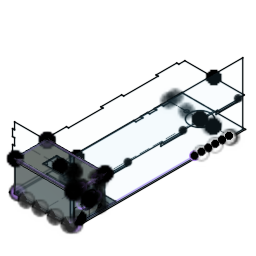
Stepper Bodies (Autodesk Fusion 360 design; units mm, degrees)
Autodesk Fusion 360 part; units mm, degrees
(part 1 of 5)
sketch "Sketch1" plane through (0, 0, 0) normal (0, 0, 1) x (1, 0, 0)
  line L0 (0, 0) -> (80, 0)
  line L1 (80, 0) -> (80, 42.25)
  line L2 (80, 42.25) -> (0, 42.25)
  line L3 (0, 42.25) -> (0, 0)
  line L4 (0, 0) -> (-2, 0) construction
  line L5 (-2, 0) -> (-2, -2) construction
  line L6 (-2, -2) -> (0, -2) construction
  line L7 (0, -2) -> (0, 0) construction
  line L8 (-2, -2) -> (82, -2)
  line L9 (82, -2) -> (82, 44.25)
  line L10 (82, 44.25) -> (-2, 44.25)
  line L11 (-2, 44.25) -> (-2, -2)
  line L12 (-2, 44.25) -> (82, 44.25) construction
  line L13 (82, 44.25) -> (82, 59.25)
  line L14 (82, 59.25) -> (-2, 59.25)
  line L15 (-2, 59.25) -> (-2, 44.25)
  line L16 (-2, 44.25) -> (82, 44.25) construction
  line L17 (82, 44.25) -> (82, 51.75) construction
  line L18 (82, 51.75) -> (-2, 51.75) construction
  line L19 (-2, 51.75) -> (-2, 44.25) construction
  circle A0 centre (40, 51.75) radius 2.5
  line L20 (40, 51.75) -> (-2, 51.75) construction
  circle A1 centre (19, 51.75) radius 2.5
  line L21 (40, 59.25) -> (40, 44.25) construction
  circle A2 centre (61, 51.75) radius 2.5
  dimension "d9" = 80
  dimension "d10" = 42.25
  dimension "d11" = 2
  dimension "d12" = 2
  dimension "d13" = 84
  dimension "d14" = 46.25
  dimension "d15" = 84
  dimension "d16" = 15
  dimension "d17" = 5
  dimension "d18" = 5
  constraint horizontal L0
  constraint vertical L1
  constraint horizontal L2
  constraint vertical L3
  constraint coincident L0.start L3.end
  constraint horizontal L4
  constraint vertical L5
  constraint horizontal L6
  constraint vertical L7
  constraint horizontal L8
  constraint vertical L9
  constraint horizontal L10
  constraint vertical L11
  constraint horizontal L12
  constraint vertical L13
  constraint horizontal L14
  constraint vertical L15
  constraint horizontal L16
  constraint vertical L17
  constraint horizontal L18
  constraint vertical L19
  constraint midpoint L13 L17.end
  constraint midpoint L18 A0.centre
  constraint coincident A0.centre L20.start
  constraint midpoint L20 A1.centre
  constraint midpoint L14 L21.start
  constraint midpoint L16 L21.end
  constraint symmetric A1 L21 A2
  measures "d9" distance of L0.start L0.end
  measures "d10" distance of L0.start L2.end
  measures "d11" distance of L0.start L4.end
  measures "d12" distance of L0.start L6.end
  measures "d13" distance of L5.end L8.end
  measures "d14" distance of L5.end L10.end
  measures "d15" distance of L10.end L9.end
  measures "d16" distance of L10.end L14.end
  measures "d17" diameter of A0
  measures "d18" diameter of A1
extrude "Extrude1" add sketch "Sketch1" along normal blind 42.25 contours L8 L9 L10 L11 makes body 1
extrude "Extrude2" add sketch "Sketch1" against normal blind 2 contours L0 L1 L2 L3 | L8 L9 L10 L11 | L10 L13 L14 L15 bodies 1
sketch "Sketch2" plane through (82, 0, 0) normal (1, 0, 0) x (0, 1, 0)
  line L0 (44.25, 0) -> (44.25, 42.25)
  line L1 (44.25, 42.25) -> (-2, 42.25)
  line L2 (-2, 42.25) -> (-2, -2)
  line L3 (-2, -2) -> (59.25, -2)
  line L4 (59.25, -2) -> (59.25, 0)
  line L5 (59.25, 0) -> (44.25, 0)
  line L6 (0, 0) -> (6, 0) construction
  line L7 (6, 0) -> (6, 6) construction
  line L8 (6, 6) -> (0, 6) construction
  line L9 (0, 6) -> (0, 0) construction
  circle A0 centre (6, 6) radius 2
  line L10 (0, 0) -> (21.125, 0) construction
  line L11 (21.125, 0) -> (21.125, 21.125) construction
  line L12 (21.125, 21.125) -> (0, 21.125) construction
  line L13 (0, 21.125) -> (0, 0) construction
  circle A1 centre (36.25, 6) radius 2
  circle A2 centre (6, 36.25) radius 2
  circle A3 centre (36.25, 36.25) radius 2
  circle A4 centre (21.125, 21.125) radius 11
  line L14 (10.125, 21.125) -> (10.125, 42.25)
  line L15 (32.125, 21.125) -> (32.125, 42.25)
  dimension "d24" = 6
  dimension "d25" = 6
  dimension "d26" = 4
  dimension "d27" = 21.125
  dimension "d28" = 21.125
  dimension "d32" = 22
  dimension "d33" = 21.125
  constraint horizontal L6
  constraint vertical L7
  constraint horizontal L8
  constraint vertical L9
  constraint coincident L6.start L9.end
  constraint coincident L7.end L8.start
  constraint horizontal L10
  constraint vertical L11
  constraint horizontal L12
  constraint vertical L13
  constraint symmetric A0 L11 A1
  constraint symmetric A0 L12 A2
  constraint symmetric L12 A1 A3
  constraint coincident L11.end L12.start
  constraint perpendicular L1 L14
  constraint coincident L12 L14.start
  constraint tangent A4 L14
  constraint symmetric L11 L14.start L15.start
  constraint symmetric L11 L14.end L15.end
  measures "d24" distance of L6.start L6.end
  measures "d25" distance of L6.start L8.end
  measures "d26" diameter of A0
  measures "d27" distance of L6.start L10.end
  measures "d28" distance of L6.start L12.end
  measures "d32" diameter of A4
  measures "d33" distance of L14.start L14.end
extrude "Extrude4" cut sketch "Sketch2" against normal blind 100 contours L1 A4 L14 L15 | A4 bodies 1
sketch "Sketch5" plane through (0, 0, 0) normal (0, 0, 1) x (1, 0, 0)
  line L0 (0, 0) -> (-6, 0) construction
  line L1 (-6, 0) -> (-6, -6) construction
  line L2 (-6, -6) -> (0, -6) construction
  line L3 (0, -6) -> (0, 0) construction
  line L4 (86, 244) -> (-6, 244)
  line L5 (-6, 244) -> (40, 244) construction
  line L6 (40, 244) -> (40, 224) construction
  line L7 (40, 224) -> (-6, 224) construction
  line L8 (-6, 224) -> (-6, 244) construction
  circle A0 centre (40, 224) radius 15
  circle A1 centre (19, 51.75) radius 2.5
  circle A2 centre (40, 51.75) radius 2.5
  circle A3 centre (61, 51.75) radius 2.5
  line L9 (-6, 224) -> (86, 224) construction
  line L10 (55, 224) -> (57, 224) construction
  circle A4 centre (59.5, 224) radius 2.5
  line L11 (57, 226.5) -> (57, 221.5) construction
  circle A5 centre (20.5, 224) radius 2.5
  circle A6 centre (19, 51.75) radius 2.5
  circle A7 centre (40, 51.75) radius 2.5
  circle A8 centre (61, 51.75) radius 2.5
  line L12 (-6, 244) -> (-6, 234) construction
  line L13 (-6, 224) -> (-3, 224)
  line L14 (-3, 224) -> (-3, 214)
  line L15 (-3, 214) -> (-6, 214)
  line L16 (-6, 244) -> (-6, 224)
  line L17 (-6, 214) -> (-6, 204) construction
  line L18 (-6, 204) -> (-3, 204)
  line L19 (-3, 204) -> (-3, 194)
  line L20 (-3, 194) -> (-6, 194)
  line L21 (-6, 214) -> (-6, 204)
  line L22 (-6, 194) -> (-6, 184) construction
  line L23 (-6, 184) -> (-3, 184)
  line L24 (-3, 184) -> (-3, 174)
  line L25 (-3, 174) -> (-6, 174)
  line L26 (-6, 194) -> (-6, 184)
  line L27 (-6, 174) -> (-6, -6)
  line L28 (-6, -6) -> (4, -6) construction
  line L29 (14, -6) -> (14, -3)
  line L30 (14, -3) -> (4, -3)
  line L31 (4, -3) -> (4, -6)
  line L32 (-6, -6) -> (4, -6)
  line L33 (14, -6) -> (24, -6) construction
  line L34 (34, -6) -> (34, -3)
  line L35 (34, -3) -> (24, -3)
  line L36 (24, -3) -> (24, -6)
  line L37 (14, -6) -> (24, -6)
  line L38 (40, 244) -> (40, -6) construction
  line L39 (76, -3) -> (76, -6)
  line L40 (66, -3) -> (76, -3)
  line L41 (66, -6) -> (66, -3)
  line L42 (56, -3) -> (56, -6)
  line L43 (46, -3) -> (56, -3)
  line L44 (46, -6) -> (46, -3)
  line L45 (34, -6) -> (46, -6)
  line L46 (56, -6) -> (66, -6)
  line L47 (76, -6) -> (86, -6)
  line L48 (83, 224) -> (83, 214)
  line L49 (83, 214) -> (86, 214)
  line L50 (86, 224) -> (83, 224)
  line L51 (86, 204) -> (83, 204)
  line L52 (83, 204) -> (83, 194)
  line L53 (83, 194) -> (86, 194)
  line L54 (86, 184) -> (83, 184)
  line L55 (83, 184) -> (83, 174)
  line L56 (83, 174) -> (86, 174)
  line L57 (86, 224) -> (86, 244)
  line L58 (86, 204) -> (86, 214)
  line L59 (86, -6) -> (86, 174)
  line L60 (86, 184) -> (86, 194)
  point P0 (40, 224)
  dimension "d40" = 6
  dimension "d41" = 6
  dimension "d44" = 92
  dimension "d45" = 250
  dimension "d47" = 46
  dimension "d48" = 20
  dimension "d50" = 30
  dimension "d52" = 2
  dimension "d53" = 5
  dimension "d54" = 5
  dimension "d55" = 5
  dimension "d56" = 5
  dimension "d57" = 5
  dimension "d60" = 10
  dimension "d61" = 3
  dimension "d62" = 10
  dimension "d63" = 10
  dimension "d64" = 3
  dimension "d65" = 10
  dimension "d92" = 10
  dimension "d93" = 3
  dimension "d94" = 10
  dimension "d95" = 10
  dimension "d96" = 10
  dimension "d97" = 3
  dimension "d98" = 10
  dimension "d99" = 10
  dimension "d100" = 3
  constraint horizontal L0
  constraint vertical L1
  constraint horizontal L2
  constraint vertical L3
  constraint coincident L0.start L3.end
  constraint horizontal L32
  constraint vertical L59
  constraint horizontal L4
  constraint vertical L16
  constraint horizontal L5
  constraint vertical L6
  constraint horizontal L7
  constraint vertical L8
  constraint coincident P0 L6.end
  constraint midpoint L9 P0
  constraint perpendicular L9 L57
  constraint coincident A0 L10.start
  constraint coincident L9 L10.start
  constraint perpendicular L10 L57
  constraint coincident L9 A4.centre
  constraint midpoint L10.end L11
  constraint perpendicular L10 L11
  constraint tangent A4 L11
  constraint symmetric L6 A4 A5
  constraint concentric A1 A6
  constraint concentric A2 A7
  constraint concentric A3 A8
  constraint perpendicular L7 L12
  constraint horizontal L13
  constraint vertical L14
  constraint horizontal L15
  constraint collinear L16 L21
  constraint perpendicular L15 L17
  constraint horizontal L18
  constraint vertical L19
  constraint horizontal L20
  constraint collinear L21 L26
  constraint perpendicular L20 L22
  constraint horizontal L23
  constraint vertical L24
  constraint horizontal L25
  constraint collinear L26 L27
  constraint perpendicular L28 L59
  constraint vertical L29
  constraint horizontal L30
  constraint vertical L31
  constraint collinear L32 L37
  constraint vertical L34
  constraint horizontal L35
  constraint vertical L36
  constraint collinear L37 L45
  constraint coincident L38.end L45
  constraint perpendicular L38 L45
  constraint symmetric L28.end L38 L39.end
  constraint symmetric L29.start L38 L41.start
  constraint symmetric L29.end L38 L40.start
  constraint symmetric L30.end L38 L39.start
  constraint symmetric L33.end L38 L42.end
  constraint symmetric L34.start L38 L44.start
  constraint symmetric L34.end L38 L43.start
  constraint symmetric L35.end L38 L42.start
  constraint collinear L45 L46
  constraint collinear L46 L47
  constraint symmetric L7.end L38 L9.end
  constraint symmetric L13.end L38 L48.start
  constraint symmetric L14.end L38 L48.end
  constraint symmetric L15.end L38 L49.end
  constraint symmetric L17.end L38 L51.start
  constraint symmetric L18.end L38 L51.end
  constraint symmetric L19.end L38 L52.end
  constraint symmetric L20.end L38 L53.end
  constraint symmetric L22.end L38 L54.start
  constraint symmetric L23.end L38 L54.end
  constraint symmetric L24.end L38 L55.end
  constraint symmetric L25.end L38 L56.end
  constraint collinear L57 L58
  constraint collinear L58 L60
  constraint collinear L59 L60
  measures "d40" distance of L0.start L0.end
  measures "d41" distance of L0.start L2.end
  measures "d44" distance of L1.end L47.end
  measures "d45" distance of L1.end L4.end
  measures "d47" distance of L4.end L5.end
  measures "d48" distance of L4.end L7.end
  measures "d50" diameter of A0
  measures "d52" distance of L10.start L10.end
  measures "d53" diameter of A4
  measures "d54" distance of L11.start L11.end
  measures "d55" diameter of A6
  measures "d56" diameter of A7
  measures "d57" diameter of A8
  measures "d60" distance of L4.end L12.end
  measures "d61" distance of L7.end L13.end
  measures "d62" distance of L7.end L15.end
  measures "d63" distance of L15.end L17.end
  measures "d64" distance of L17.end L18.end
  measures "d65" distance of L17.end L20.end
  measures "d92" distance of L20.end L22.end
  measures "d93" distance of L22.end L23.end
  measures "d94" distance of L22.end L25.end
  measures "d95" distance of L1.end L28.end
  measures "d96" distance of L28.end L29.start
  measures "d97" distance of L28.end L30.end
  measures "d98" distance of L29.start L33.end
  measures "d99" distance of L33.end L34.start
  measures "d100" distance of L33.end L35.end
ref_plane "WorkPlane2" through (40, 21.125, 42.25) normal (0, 0, 1) x (1, 0, 0)
sketch "Sketch6" plane through (0, 0, 42.25) normal (0, 0, 1) x (1, 0, 0)
  line L0 (-2, 44.25) -> (82, 44.25)
  line L1 (-2, 44.25) -> (-2, -2)
  line L2 (-2, -2) -> (82, -2)
  line L3 (82, 10.125) -> (82, 32.125)
  line L4 (82, -2) -> (82, 44.25)
  line L5 (82, 4) -> (82, 8)
  line L6 (-2, 44.25) -> (-3, 44.25) construction
  line L7 (-3, 44.25) -> (-3, 45.25) construction
  line L8 (-3, 45.25) -> (-2, 45.25) construction
  line L9 (-2, 45.25) -> (-2, 44.25) construction
  line L10 (-2, -2) -> (-3, -2) construction
  line L11 (-3, -2) -> (-3, -3) construction
  line L12 (-3, -3) -> (-2, -3) construction
  line L13 (-2, -3) -> (-2, -2) construction
  line L14 (82, -2) -> (83, -2) construction
  line L15 (83, -2) -> (83, -3) construction
  line L16 (83, -3) -> (82, -3) construction
  line L17 (82, -3) -> (82, -2) construction
  line L18 (82, 44.25) -> (83, 44.25) construction
  line L19 (83, 44.25) -> (83, 45.25) construction
  line L20 (83, 45.25) -> (82, 45.25) construction
  line L21 (82, 45.25) -> (82, 44.25) construction
  line L22 (-3, 45.25) -> (83, 45.25)
  line L23 (83, 45.25) -> (83, -3)
  line L24 (83, -3) -> (-3, -3)
  line L25 (-3, -3) -> (-3, 45.25)
  line L26 (-2, 44.25) -> (82, 44.25)
  line L27 (82, 44.25) -> (82, -2)
  line L28 (82, -2) -> (-2, -2)
  line L29 (-2, -2) -> (-2, 44.25)
  line L30 (-2, 21.125) -> (82, 21.125) construction
  line L31 (40, 44.25) -> (40, -2) construction
  line L32 (55, 31.125) -> (25, 31.125)
  line L33 (25, 31.125) -> (25, 11.125)
  line L34 (25, 11.125) -> (55, 11.125)
  line L35 (55, 11.125) -> (55, 31.125)
  line L36 (55, 31.125) -> (25, 11.125) construction
  line L37 (25, 31.125) -> (55, 11.125) construction
  point P0 (82, 36.25)
  point P1 (82, 6)
  point P2 (40, 21.125)
  dimension "d68" = 1
  dimension "d69" = 1
  dimension "d70" = 1
  dimension "d71" = 1
  dimension "d72" = 1
  dimension "d73" = 1
  dimension "d74" = 1
  dimension "d75" = 1
  dimension "d86" = 30
  dimension "d87" = 20
  constraint horizontal L6
  constraint vertical L7
  constraint horizontal L8
  constraint vertical L9
  constraint coincident L0.start L1.start
  constraint horizontal L10
  constraint vertical L11
  constraint horizontal L12
  constraint vertical L13
  constraint coincident L1.end L2.start
  constraint horizontal L14
  constraint vertical L15
  constraint horizontal L16
  constraint vertical L17
  constraint coincident L2.end L4.start
  constraint horizontal L18
  constraint vertical L19
  constraint horizontal L20
  constraint vertical L21
  constraint coincident L0.end L4.end
  constraint horizontal L22
  constraint vertical L23
  constraint horizontal L24
  constraint vertical L25
  constraint horizontal L26
  constraint vertical L27
  constraint horizontal L28
  constraint vertical L29
  constraint midpoint L1 L30.start
  constraint midpoint L4 L30.end
  constraint midpoint L0 L31.start
  constraint midpoint L28 L31.end
  constraint horizontal L32
  constraint perpendicular L32 L33
  constraint parallel L32 L34
  constraint parallel L33 L35
  constraint coincident L36 P2
  constraint coincident L37 P2
  constraint midpoint L31 P2
  measures "d68" distance of L0.start L6.end
  measures "d69" distance of L0.start L8.end
  measures "d70" distance of L1.end L10.end
  measures "d71" distance of L1.end L12.end
  measures "d72" distance of L2.end L14.end
  measures "d73" distance of L2.end L16.end
  measures "d74" distance of L0.end L18.end
  measures "d75" distance of L0.end L20.end
  measures "d86" distance of L33.end L34.end
  measures "d87" distance of L32.end L33.end
extrude "Extrude6" add sketch "Sketch6" against normal blind 3 contours L22 L23 L24 L25 bodies 1
extrude "Extrude7" add sketch "Sketch6" against normal blind 3 separate body contours L22 L23 L24 L25 makes body 2
extrude "Extrude10" add sketch "Sketch6" along normal blind 1 contours L0 L1 L2 L3 L4 L5 L26 L27 L28 L29 | L22 L23 L24 L25 bodies 2
sketch "Sketch8" plane through (82, 0, 0) normal (1, 0, 0) x (0, 1, 0)
  line L0 (44.25, 39.25) -> (32.125, 39.25)
  line L1 (32.125, 39.25) -> (32.125, 21.125)
  arc A0 (10.125, 21.125) -> (32.125, 21.125) centre (21.125, 21.125) ccw
  line L2 (10.125, 21.125) -> (10.125, 39.25)
  line L3 (10.125, 39.25) -> (-2, 39.25)
  line L4 (-2, 39.25) -> (-2, -2)
  line L5 (-2, -2) -> (59.25, -2)
  line L6 (59.25, -2) -> (59.25, 0)
  line L7 (59.25, 0) -> (44.25, 0)
  line L8 (44.25, 0) -> (44.25, 39.25)
  line L9 (-6, 0) -> (174, 0)
  line L10 (-6, 0) -> (-6, -2) construction
  line L11 (244, -2) -> (244, 88)
  line L12 (244, 88) -> (-6, 88)
  line L13 (45.25, 39.25) -> (-3, 39.25)
  line L14 (-3, 39.25) -> (-6, 39.25) construction
  line L15 (45.25, 39.25) -> (75.25, 39.25)
  line L16 (75.25, 39.25) -> (75.25, 36.25)
  line L17 (75.25, 36.25) -> (45.25, 36.25)
  line L18 (45.25, 36.25) -> (45.25, 39.25)
  line L19 (125.25, 39.25) -> (155.25, 39.25)
  line L20 (125.25, 36.25) -> (125.25, 39.25)
  line L21 (155.25, 36.25) -> (125.25, 36.25)
  line L22 (155.25, 39.25) -> (155.25, 36.25)
  line L23 (205.25, 39.25) -> (235.25, 39.25)
  line L24 (205.25, 36.25) -> (205.25, 39.25)
  line L25 (235.25, 36.25) -> (205.25, 36.25)
  line L26 (235.25, 39.25) -> (235.25, 36.25)
  arc A1 (10.125, 21.125) -> (32.125, 21.125) centre (21.125, 21.125) ccw
  circle A2 centre (21.125, 21.125) radius 11
  line L27 (174, 0) -> (174, -2) construction
  line L28 (184, 0) -> (184, -2) construction
  line L29 (194, 0) -> (194, -2) construction
  line L30 (204, 0) -> (204, -2) construction
  line L31 (214, 0) -> (214, -2) construction
  line L32 (224, 0) -> (224, -2) construction
  line L33 (184, -2) -> (184, -5)
  line L34 (184, -5) -> (174, -5)
  line L35 (174, -5) -> (174, -2)
  line L36 (-6, -2) -> (174, -2)
  line L37 (204, -2) -> (204, -5)
  line L38 (204, -5) -> (194, -5)
  line L39 (194, -5) -> (194, -2)
  line L40 (184, -2) -> (194, -2)
  line L41 (224, -2) -> (224, -5)
  line L42 (224, -5) -> (214, -5)
  line L43 (214, -5) -> (214, -2)
  line L44 (204, -2) -> (214, -2)
  line L45 (224, -2) -> (244, -2)
  line L46 (-6, 88) -> (-6, 78) construction
  line L47 (-6, 78) -> (-3, 78)
  line L48 (-3, 78) -> (-3, 68)
  line L49 (-3, 68) -> (-6, 68)
  line L50 (-6, 88) -> (-6, 78)
  line L51 (-6, 68) -> (-6, 58) construction
  line L52 (-6, 58) -> (-3, 58)
  line L53 (-3, 58) -> (-3, 48)
  line L54 (-3, 48) -> (-6, 48)
  line L55 (-6, 68) -> (-6, 58)
  line L56 (-6, 48) -> (-6, -2)
  point P0 (174, 0)
  point P1 (184, 0)
  point P2 (194, 0)
  point P3 (204, 0)
  point P4 (224, 0)
  point P5 (214, 0)
  dimension "d103" = 2
  dimension "d104" = 250
  dimension "d105" = 90
  dimension "d107" = 30
  dimension "d108" = 3
  dimension "d111" = 160
  dimension "d112" = 0
  dimension "d113" = 22
  dimension "d114" = 10
  dimension "d115" = 3
  dimension "d116" = 10
  dimension "d117" = 3
  dimension "d118" = 10
  dimension "d119" = 3
  dimension "d120" = 10
  dimension "d121" = 3
  dimension "d122" = 10
  dimension "d123" = 10
  dimension "d124" = 3
  dimension "d125" = 10
  constraint coincident L9.start L10.start
  constraint perpendicular L9 L10
  constraint horizontal L36
  constraint vertical L11
  constraint horizontal L12
  constraint vertical L50
  constraint coincident L13.end L14.start
  constraint coincident L14.end L56
  constraint perpendicular L14 L56
  constraint horizontal L15
  constraint vertical L16
  constraint horizontal L17
  constraint vertical L18
  constraint coincident L13.start L15.start
  constraint concentric A1 A2
  constraint coincident P0 L9.end
  constraint perpendicular L27 L36
  constraint coincident P1 L28.start
  constraint perpendicular L28 L40
  constraint coincident P2 L29.start
  constraint perpendicular L29 L40
  constraint coincident P3 L30.start
  constraint perpendicular L30 L44
  constraint coincident P5 L31.start
  constraint perpendicular L31 L44
  constraint coincident P4 L32.start
  constraint perpendicular L32 L45
  constraint vertical L33
  constraint horizontal L34
  constraint vertical L35
  constraint collinear L36 L40
  constraint vertical L37
  constraint horizontal L38
  constraint vertical L39
  constraint collinear L40 L44
  constraint vertical L41
  constraint horizontal L42
  constraint vertical L43
  constraint collinear L44 L45
  constraint perpendicular L12 L46
  constraint horizontal L47
  constraint vertical L48
  constraint horizontal L49
  constraint collinear L50 L55
  constraint horizontal L52
  constraint vertical L53
  constraint horizontal L54
  constraint collinear L55 L56
  measures "d103" distance of L9.start L10.end
  measures "d104" distance of L10.end L11.start
  measures "d105" distance of L10.end L12.end
  measures "d107" distance of L13.start L15.end
  measures "d108" distance of L13.start L17.end
  measures "d113" diameter of A2
  measures "d114" distance of L27.end L28.end
  measures "d115" distance of L27.end L34.end
  measures "d116" distance of L29.end L30.end
  measures "d117" distance of L29.end L38.end
  measures "d118" distance of L31.end L32.end
  measures "d119" distance of L31.end L42.end
  measures "d120" distance of L12.end L46.end
  measures "d121" distance of L46.end L47.end
  measures "d122" distance of L46.end L49.end
  measures "d123" distance of L49.end L51.end
  measures "d124" distance of L51.end L52.end
  measures "d125" distance of L51.end L54.end
sketch "Sketch10" plane through (0, -2, 0) normal (0, -1, 0) x (1, 0, 0)
  line L0 (82, 39.25) -> (-2, 39.25)
  line L1 (-2, 39.25) -> (-2, -2)
  line L2 (-2, -2) -> (82, -2)
  line L3 (82, -2) -> (82, 39.25)
  line L4 (-6, 0) -> (4, 0)
  line L5 (14, 0) -> (24, 0)
  line L6 (34, 0) -> (46, 0)
  line L7 (56, 0) -> (66, 0)
  line L8 (-6, 0) -> (-3, 0) construction
  line L9 (86, 0) -> (83, 0) construction
  line L10 (82, -2) -> (83, -2) construction
  line L11 (83, 0) -> (83, -10.8119) construction
  line L12 (82, 88) -> (-10, 88) construction
  line L13 (-3, 88) -> (83, 88)
  line L14 (76, 0) -> (86, 0)
  line L15 (4, 0) -> (4, -2) construction
  line L16 (14, 0) -> (14, -2) construction
  line L17 (24, 0) -> (24, -2) construction
  line L18 (34, 0) -> (34, -2) construction
  line L19 (46, 0) -> (46, -2) construction
  line L20 (56, 0) -> (56, -2) construction
  line L21 (66, 0) -> (66, -2) construction
  line L22 (76, 0) -> (76, -2) construction
  line L23 (14, -2) -> (14, -5)
  line L24 (14, -5) -> (4, -5)
  line L25 (4, -5) -> (4, -2)
  line L26 (4, -2) -> (-3, -2)
  line L27 (34, -2) -> (34, -5)
  line L28 (34, -5) -> (24, -5)
  line L29 (24, -5) -> (24, -2)
  line L30 (24, -2) -> (14, -2)
  line L31 (56, -2) -> (56, -5)
  line L32 (56, -5) -> (46, -5)
  line L33 (46, -5) -> (46, -2)
  line L34 (46, -2) -> (34, -2)
  line L35 (76, -2) -> (76, -5)
  line L36 (76, -5) -> (66, -5)
  line L37 (66, -5) -> (66, -2)
  line L38 (83, -2) -> (76, -2)
  line L39 (66, -2) -> (56, -2)
  line L40 (82, 78) -> (82, 68)
  line L41 (82, 58) -> (82, 48)
  line L42 (82, 78) -> (83, 78) construction
  line L43 (82, 68) -> (83, 68) construction
  line L44 (82, 58) -> (83, 58) construction
  line L45 (82, 48) -> (83, 48) construction
  line L46 (83, 78) -> (86, 78)
  line L47 (86, 78) -> (86, 68)
  line L48 (86, 68) -> (83, 68)
  line L49 (83, 88) -> (83, 78)
  line L50 (83, 58) -> (86, 58)
  line L51 (86, 58) -> (86, 48)
  line L52 (86, 48) -> (83, 48)
  line L53 (83, 68) -> (83, 58)
  line L54 (83, 48) -> (83, -2)
  line L55 (40, 88) -> (40, -19.3098) construction
  line L56 (-3, 78) -> (-6, 78)
  line L57 (-6, 78) -> (-6, 68)
  line L58 (-6, 68) -> (-3, 68)
  line L59 (-3, 58) -> (-6, 58)
  line L60 (-6, 58) -> (-6, 48)
  line L61 (-6, 48) -> (-3, 48)
  line L62 (-3, 78) -> (-3, 88)
  line L63 (-3, -2) -> (-3, 48)
  line L64 (-3, 58) -> (-3, 68)
  point P0 (86, 0)
  point P1 (82, -2)
  point P2 (82, 88)
  dimension "d126" = 3
  dimension "d127" = 3
  dimension "d128" = 92
  dimension "d129" = 10
  dimension "d130" = 3
  dimension "d131" = 10
  dimension "d132" = 3
  dimension "d133" = 10
  dimension "d134" = 3
  dimension "d135" = 10
  dimension "d136" = 3
  dimension "d137" = 3
  dimension "d138" = 10
  dimension "d139" = 3
  dimension "d140" = 10
  constraint coincident L4.start L8.start
  constraint perpendicular L1 L8
  constraint coincident P0 L9.start
  constraint perpendicular L3 L9
  constraint coincident P1 L2.end
  constraint perpendicular L3 L10
  constraint perpendicular L10 L11
  constraint coincident L10.end L11
  constraint coincident P2 L12.start
  constraint horizontal L12
  constraint horizontal L38
  constraint vertical L63
  constraint horizontal L13
  constraint vertical L49
  constraint coincident L12 L13.start
  constraint coincident L8.end L63
  constraint coincident L4.end L15.start
  constraint perpendicular L15 L26
  constraint coincident L5.start L16.start
  constraint perpendicular L2 L16
  constraint coincident L5.end L17.start
  constraint perpendicular L17 L30
  constraint coincident L6.start L18.start
  constraint perpendicular L18 L34
  constraint coincident L6.end L19.start
  constraint perpendicular L19 L34
  constraint coincident L7.start L20.start
  constraint perpendicular L20 L39
  constraint coincident L7.end L21.start
  constraint perpendicular L21 L39
  constraint coincident L14.start L22.start
  constraint perpendicular L22 L38
  constraint vertical L23
  constraint horizontal L24
  constraint vertical L25
  constraint collinear L26 L30
  constraint vertical L27
  constraint horizontal L28
  constraint vertical L29
  constraint collinear L30 L34
  constraint vertical L31
  constraint horizontal L32
  constraint vertical L33
  constraint collinear L34 L39
  constraint vertical L35
  constraint horizontal L36
  constraint vertical L37
  constraint collinear L38 L39
  constraint coincident L40.start L42.start
  constraint perpendicular L42 L49
  constraint coincident L40.end L43.start
  constraint perpendicular L43 L53
  constraint coincident L41.start L44.start
  constraint perpendicular L44 L53
  constraint coincident L41.end L45.start
  constraint perpendicular L45 L54
  constraint horizontal L46
  constraint vertical L47
  constraint horizontal L48
  constraint collinear L49 L53
  constraint horizontal L50
  constraint vertical L51
  constraint horizontal L52
  constraint collinear L53 L54
  constraint midpoint L13 L55.start
  constraint perpendicular L34 L55
  constraint symmetric L42.end L55 L56.start
  constraint symmetric L44.end L55 L59.start
  constraint symmetric L46.end L55 L56.end
  constraint symmetric L47.end L55 L57.end
  constraint symmetric L43.end L55 L58.end
  constraint symmetric L50.end L55 L59.end
  constraint symmetric L51.end L55 L60.end
  constraint symmetric L45.end L55 L61.end
  constraint collinear L62 L64
  constraint collinear L63 L64
  measures "d126" distance of L4.start L8.end
  measures "d127" distance of P0 L9.end
  measures "d128" distance of P2 L12.end
  measures "d129" distance of L15.end L16.end
  measures "d130" distance of L15.end L24.end
  measures "d131" distance of L17.end L18.end
  measures "d132" distance of L17.end L28.end
  measures "d133" distance of L19.end L20.end
  measures "d134" distance of L19.end L32.end
  measures "d135" distance of L21.end L22.end
  measures "d136" distance of L21.end L36.end
  measures "d137" distance of L42.end L46.end
  measures "d138" distance of L42.end L43.end
  measures "d139" distance of L44.end L50.end
  measures "d140" distance of L44.end L45.end
sketch "CF349-3" plane through (0, 0, 0) normal (0, 1, 0) x (1, 0, 0)
  ellipse E0 centre (9.7927, -31.8351) end of major axis (9.5411, -31.8891) minor radius 0.1979 (10.029, -31.89) -> (10.0412, -31.8585) ccw
  ellipse E1 centre (12.0374, -31.8103) end of major axis (10.491, -33.8583) minor radius 1.787 (10.29, -31.2409) -> (10.0412, -31.8585) ccw
  spline S0 degree 3 poles (10.29, -31.2409) (10.3575, -31.1119) (10.4304, -30.9612) (10.5094, -30.7977) (10.922, -29.9448) (11.5452, -28.6559) (12.4109, -28.5567) knots 2 2 2 2 3 3 3 4 4 4 4
  spline S1 degree 3 poles (12.4109, -28.5567) (13.6884, -28.4121) (15.0142, -29.6655) (15.9809, -30.5824) knots 4 4 4 4 5 5 5 5
  spline S2 degree 3 poles (15.9809, -30.5824) (16.0708, -30.6676) (16.1573, -30.7496) (16.24, -30.827) knots 5 5 5 5 6 6 6 6
  spline S3 degree 3 poles (16.24, -30.827) (16.3502, -30.9302) (16.461, -31.0304) (16.5719, -31.1284) knots 6 6 6 6 7 7 7 7
  spline S4 degree 3 poles (16.5719, -31.1284) (16.6214, -31.1722) (16.6713, -31.2147) (16.7213, -31.2573) knots 7 7 7 7 8 8 8 8
  line L0 (16.7213, -31.2573) -> (16.773, -31.3012)
  spline S5 degree 3 poles (16.773, -31.3012) (16.8143, -31.3372) (16.856, -31.3734) (16.8973, -31.408) knots 9 9 9 9 10 10 10 10
  spline S6 degree 3 poles (16.8973, -31.408) (16.9869, -31.4833) (17.0773, -31.557) (17.1771, -31.6376) knots 10 10 10 10 11 11 11 11
  line L1 (17.1771, -31.6376) -> (17.2167, -31.6696)
  spline S7 degree 3 poles (17.2167, -31.6696) (17.3178, -31.7506) (17.4196, -31.8305) (17.5304, -31.9155) knots 12 12 12 12 13 13 13 13
  spline S8 degree 3 poles (17.5304, -31.9155) (17.5307, -31.9157) (17.5308, -31.916) (17.531, -31.9162) knots 13 13 13 13 14 14 14 14
  spline S9 degree 3 poles (17.531, -31.9162) (17.7632, -32.0949) (18.0123, -32.2784) (18.3146, -32.4937) knots 14 14 14 14 15 15 15 15
  line L2 (18.3146, -32.4937) -> (18.3641, -32.5306)
  spline S10 degree 3 poles (18.3641, -32.5306) (18.6188, -32.7108) (18.8943, -32.9006) (19.231, -33.1274) knots 16 16 16 16 17 17 17 17
  spline S11 degree 3 poles (19.231, -33.1274) (19.4107, -33.2486) (19.5936, -33.365) (19.7764, -33.4814) knots 17 17 17 17 18 18 18 18
  spline S12 degree 3 poles (19.7764, -33.4814) (19.9104, -33.5668) (20.0444, -33.652) (20.1772, -33.7393) knots 18 18 18 18 19 19 19 19
  line L3 (20.1772, -33.7393) -> (20.2453, -33.784)
  spline S13 degree 3 poles (20.2453, -33.784) (20.873, -34.1957) (21.522, -34.6215) (22.0744, -35.132) knots 20 20 20 20 21 21 21 21
  spline S14 degree 3 poles (22.0744, -35.132) (22.2396, -35.2847) (22.431, -35.4681) (22.5996, -35.6733) knots 21 21 21 21 22 22 22 22
  spline S15 degree 3 poles (22.5996, -35.6733) (22.6008, -35.675) (22.6022, -35.6766) (22.6036, -35.6783) knots 22 22 22 22 23 23 23 23
  spline S16 degree 3 poles (22.6036, -35.6783) (22.64, -35.7224) (22.6746, -35.7677) (22.708, -35.8131) knots 23 23 23 23 24 24 24 24
  spline S17 degree 3 poles (22.708, -35.8131) (22.7523, -35.8741) (22.7957, -35.9354) (22.8348, -36.0018) knots 24 24 24 24 25 25 25 25
  spline S18 degree 3 poles (22.8348, -36.0018) (22.8809, -36.0801) (22.9252, -36.1608) (22.9696, -36.2418) knots 25 25 25 25 26 26 26 26
  spline S19 degree 3 poles (22.9696, -36.2418) (23.1062, -36.4904) (23.2473, -36.7475) (23.4499, -36.9562) knots 26 26 26 26 27 27 27 27
  spline S20 degree 3 poles (23.4499, -36.9562) (23.8134, -37.3311) (24.1811, -37.7086) (24.5639, -38.0957) knots 27 27 27 27 28 28 28 28
  spline S21 degree 3 poles (24.5639, -38.0957) (24.5675, -38.1002) (24.5714, -38.1045) (24.5756, -38.1086) knots 28 28 28 28 29 29 29 29
  spline S22 degree 3 poles (24.5756, -38.1086) (24.9707, -38.5086) (25.3291, -38.8639) (25.6692, -39.1925) knots 29 29 29 29 30 30 30 30
  spline S23 degree 3 poles (25.6692, -39.1925) (25.6609, -39.243) (25.6521, -39.2939) (25.6425, -39.3453) knots 30 30 30 30 31 31 31 31
  spline S24 degree 3 poles (25.6425, -39.3453) (25.6369, -39.3755) (25.632, -39.4052) (25.626, -39.4356) knots 31 31 31 31 32 32 32 32
  spline S25 degree 3 poles (25.626, -39.4356) (25.6094, -39.5205) (25.5908, -39.6064) (25.5713, -39.6927) knots 32 32 32 32 33 33 33 33
  spline S26 degree 3 poles (25.5713, -39.6927) (25.5682, -39.7058) (25.5658, -39.7188) (25.5628, -39.7319) knots 33 33 33 33 34 34 34 34
  spline S27 degree 3 poles (25.5628, -39.7319) (25.5627, -39.7323) (25.5627, -39.7326) (25.5626, -39.733) knots 34 34 34 34 35 35 35 35
  line L4 (25.5626, -39.733) -> (25.538, -39.8435)
  spline S28 degree 3 poles (25.538, -39.8435) (25.5237, -39.9005) (25.5076, -39.9567) (25.4916, -40.0131) knots 36 36 36 36 37 37 37 37
  line L5 (25.4916, -40.0131) -> (25.4787, -40.0588)
  spline S29 degree 3 poles (25.4787, -40.0588) (25.4627, -40.1173) (25.4467, -40.1764) (25.4288, -40.2342) knots 38 38 38 38 39 39 39 39
  spline S30 degree 3 poles (25.4288, -40.2342) (25.4089, -40.2982) (25.3874, -40.3616) (25.3659, -40.4244) knots 39 39 39 39 40 40 40 40
  spline S31 degree 3 poles (25.3659, -40.4244) (25.3437, -40.4896) (25.3206, -40.5545) (25.2961, -40.6185) knots 40 40 40 40 41 41 41 41
  spline S32 degree 3 poles (25.2961, -40.6185) (25.2742, -40.6766) (25.2515, -40.7342) (25.2283, -40.791) knots 41 41 41 41 42 42 42 42
  spline S33 degree 3 poles (25.2283, -40.791) (25.1993, -40.8608) (25.1685, -40.9299) (25.1375, -40.9979) knots 42 42 42 42 43 43 43 43
  line L6 (25.1375, -40.9979) -> (25.119, -41.038)
  spline S34 degree 3 poles (25.119, -41.038) (25.1016, -41.0759) (25.0841, -41.1139) (25.066, -41.1511) knots 44 44 44 44 45 45 45 45
  spline S35 degree 3 poles (25.066, -41.1511) (25.0277, -41.2285) (24.9859, -41.3048) (24.9439, -41.3811) knots 45 45 45 45 46 46 46 46
  line L7 (24.9439, -41.3811) -> (24.9204, -41.4243)
  spline S36 degree 3 poles (24.9204, -41.4243) (24.9063, -41.4503) (24.8924, -41.4764) (24.8775, -41.5018) knots 47 47 47 47 48 48 48 48
  spline S37 degree 3 poles (24.8775, -41.5018) (24.8035, -41.6279) (24.7327, -41.7391) (24.6617, -41.8413) knots 48 48 48 48 49 49 49 49
  ellipse E2 centre (22.0709, -42.2011) end of major axis (19.0417, -44.5726) minor radius 1.6241 (24.0681, -42.5699) -> (24.6617, -41.8413) ccw
  line L8 (24.0681, -42.5699) -> (23.9134, -42.7367)
  spline S38 degree 3 poles (23.9134, -42.7367) (23.7734, -42.8877) (23.6332, -43.0392) (23.4923, -43.1848) knots 51 51 51 51 52 52 52 52
  spline S39 degree 3 poles (23.4923, -43.1848) (23.4857, -43.1916) (23.4808, -43.1997) (23.4754, -43.2075) knots 52 52 52 52 53 53 53 53
  line L9 (23.4754, -43.2075) -> (22.8589, -42.7667)
  spline S40 degree 3 poles (22.8589, -42.7667) (22.723, -42.6702) (22.5864, -42.5745) (22.45, -42.4789) knots 54 54 54 54 55 55 55 55
  line L10 (22.45, -42.4789) -> (22.183, -42.291)
  spline S41 degree 3 poles (22.183, -42.291) (22.0698, -42.2109) (21.9564, -42.1307) (21.8421, -42.0515) knots 56 56 56 56 57 57 57 57
  spline S42 degree 3 poles (21.8421, -42.0515) (21.6691, -41.932) (21.4945, -41.8148) (21.3196, -41.6976) knots 57 57 57 57 58 58 58 58
  line L11 (21.3196, -41.6976) -> (21.0848, -41.539)
  spline S43 degree 3 poles (21.0848, -41.539) (20.998, -41.4797) (20.911, -41.4205) (20.8228, -41.3624) knots 59 59 59 59 60 60 60 60
  spline S44 degree 3 poles (20.8228, -41.3624) (20.4525, -41.119) (20.1125, -40.9033) (19.7833, -40.7029) knots 60 60 60 60 61 61 61 61
  spline S45 degree 3 poles (19.7833, -40.7029) (19.7774, -40.6993) (19.7716, -40.6962) (19.7655, -40.6934) knots 61 61 61 61 62 62 62 62
  spline S46 degree 3 poles (19.7655, -40.6934) (19.333, -40.4934) (18.8545, -40.2833) (18.3145, -40.0552) knots 62 62 62 62 63 63 63 63
  ellipse E3 centre (15.6063, -39.9575) end of major axis (18.223, -36.7955) minor radius 2.3471 (18.3145, -40.0552) -> (18.7113, -38.9051) ccw
  ellipse E4 centre (17.7423, -38.1876) end of major axis (17.9324, -35.8274) minor radius 1.0627 (18.7113, -38.9051) -> (18.7797, -37.2446) ccw
  spline S47 degree 3 poles (18.7797, -37.2446) (18.7275, -36.8445) (18.3317, -36.5395) (17.9172, -36.58) knots 65 65 65 65 66 66 66 66
  spline S48 degree 3 poles (17.9172, -36.58) (17.4191, -36.6286) (17.0758, -37.073) (16.825, -37.3975) knots 66 66 66 66 67 67 67 67
  spline S49 degree 3 poles (16.825, -37.3975) (16.7935, -37.4384) (16.763, -37.4777) (16.7335, -37.5149) knots 67 67 67 67 68 68 68 68
  spline S50 degree 3 poles (16.7335, -37.5149) (16.6811, -37.5807) (16.6293, -37.6475) (16.5774, -37.7144) (16.2913, -38.0837) (16.0211, -38.4326) (15.6247, -38.6392) (15.576, -38.6646) (15.5408, -38.6782) (15.5169, -38.6854) knots 68 68 68 68 69 69 69 70 70 70 71 71 71 71
  ellipse E5 centre (15.7154, -38.3801) end of major axis (15.5407, -38.7694) minor radius 0.1044 (15.5592, -38.4934) -> (15.5169, -38.6854) ccw
  spline S51 degree 3 poles (15.5592, -38.4934) (15.7263, -37.9859) (16.1225, -37.617) (16.4488, -37.3526) knots 72 72 72 72 73 73 73 73
  spline S52 degree 3 poles (16.4488, -37.3526) (16.5361, -37.282) (16.6369, -37.2206) (16.7437, -37.1555) knots 73 73 73 73 74 74 74 74
  spline S53 degree 3 poles (16.7437, -37.1555) (16.9426, -37.0345) (17.1483, -36.9094) (17.2966, -36.7064) (17.4499, -36.4966) (17.4888, -36.1838) (17.391, -35.946) knots 74 74 74 74 75 75 75 76 76 76 76
  ellipse E6 centre (16.2442, -36.716) end of major axis (15.2224, -37.6813) minor radius 0.9268 (17.391, -35.946) -> (16.8686, -35.5505) ccw
  spline S54 degree 3 poles (16.8686, -35.5505) (16.709, -35.525) (16.5542, -35.5132) (16.4038, -35.5132) knots 77 77 77 77 78 78 78 78
  spline S55 degree 3 poles (16.4038, -35.5132) (15.5517, -35.5133) (14.8499, -35.8894) (14.3145, -36.2374) knots 78 78 78 78 79 79 79 79
  spline S56 degree 3 poles (14.3145, -36.2374) (14.2327, -36.2905) (14.1473, -36.3446) (14.0598, -36.3998) knots 79 79 79 79 80 80 80 80
  spline S57 degree 3 poles (14.0598, -36.3998) (13.5501, -36.7216) (12.9458, -37.1043) (12.5979, -37.6437) knots 80 80 80 80 81 81 81 81
  spline S58 degree 3 poles (12.5979, -37.6437) (12.3305, -37.5153) (12.0909, -37.3959) (11.8728, -37.2819) knots 81 81 81 81 82 82 82 82
  spline S59 degree 3 poles (11.8728, -37.2819) (10.876, -36.7606) (9.8144, -36.0875) (9.4983, -35.047) knots 82 82 82 82 83 83 83 83
  spline S60 degree 3 poles (9.4983, -35.047) (9.2241, -34.1434) (9.3927, -33.1401) (10.029, -31.89) knots 83 83 83 83 84 84 84 84
  spline S61 degree 3 poles (19.9343, -28.4931) (21.0931, -26.8369) (22.3738, -25.3801) (23.7298, -23.8377) knots 0 0 0 0 1 1 1 1
  spline S62 degree 3 poles (23.7298, -23.8377) (23.9918, -23.5399) (24.2543, -23.2412) (24.5165, -22.9405) knots 1 1 1 1 2 2 2 2
  spline S63 degree 3 poles (24.5165, -22.9405) (25.1132, -22.2573) (25.641, -21.4853) (26.1486, -20.7284) knots 2 2 2 2 3 3 3 3
  spline S64 degree 3 poles (26.1486, -20.7284) (25.7958, -22.4239) (25.3052, -25.6168) (25.2234, -26.8031) knots 3 3 3 3 4 4 4 4
  spline S65 degree 3 poles (25.2234, -26.8031) (25.1332, -28.1131) (25.4555, -32.0621) (25.574, -33.4337) knots 4 4 4 4 5 5 5 5
  ellipse E7 centre (26.4374, -36.4373) end of major axis (21.0331, -39.4664) minor radius 3.0628 (25.574, -33.4337) -> (24.2119, -34.2069) ccw
  ellipse E8 centre (22.6089, -36.3889) end of major axis (19.0869, -39.3426) minor radius 0.7827 (24.2119, -34.2069) -> (23.8356, -34.4608) ccw
  line L12 (23.8356, -34.4608) -> (23.7662, -34.5089)
  spline S66 degree 3 poles (23.7662, -34.5089) (23.3767, -34.7812) (23.0434, -35.0444) (22.7523, -35.3097) knots 8 8 8 8 9 9 9 9
  spline S67 degree 3 poles (22.7523, -35.3097) (22.6041, -35.1455) (22.4503, -34.999) (22.3139, -34.873) knots 9 9 9 9 10 10 10 10
  spline S68 degree 3 poles (22.3139, -34.873) (21.7401, -34.3425) (21.0785, -33.9086) (20.4389, -33.489) knots 10 10 10 10 11 11 11 11
  line L13 (20.4389, -33.489) -> (20.3708, -33.4444)
  spline S69 degree 3 poles (20.3708, -33.4444) (20.2368, -33.3563) (20.1013, -33.2701) (19.9659, -33.1838) knots 12 12 12 12 13 13 13 13
  spline S70 degree 3 poles (19.9659, -33.1838) (19.7855, -33.069) (19.6053, -32.9543) (19.4281, -32.8349) knots 13 13 13 13 14 14 14 14
  spline S71 degree 3 poles (19.4281, -32.8349) (19.0937, -32.6096) (18.8204, -32.4214) (18.5704, -32.2444) knots 14 14 14 14 15 15 15 15
  line L14 (18.5704, -32.2444) -> (18.5203, -32.2071)
  spline S72 degree 3 poles (18.5203, -32.2071) (18.5201, -32.207) (18.52, -32.2068) (18.5198, -32.2067) knots 16 16 16 16 17 17 17 17
  spline S73 degree 3 poles (18.5198, -32.2067) (18.2729, -32.031) (18.0625, -31.877) (17.8676, -31.7295) knots 17 17 17 17 18 18 18 18
  spline S74 degree 3 poles (17.8676, -31.7295) (18.4407, -30.7217) (19.1179, -29.6615) (19.9343, -28.4931) knots 18 18 18 18 19 19 19 19
  spline S75 degree 3 poles (24.8279, -37.8622) (24.8271, -37.8613) (24.8262, -37.8604) (24.8253, -37.8595) knots 0 0 0 0 1 1 1 1
  spline S76 degree 3 poles (24.8253, -37.8595) (24.4476, -37.4766) (24.0731, -37.0922) (23.7031, -36.7106) knots 1 1 1 1 2 2 2 2
  spline S77 degree 3 poles (23.7031, -36.7106) (23.5338, -36.5359) (23.4099, -36.3105) (23.2788, -36.072) knots 2 2 2 2 3 3 3 3
  spline S78 degree 3 poles (23.2788, -36.072) (23.2327, -35.9878) (23.1867, -35.904) (23.1386, -35.8225) knots 3 3 3 3 4 4 4 4
  spline S79 degree 3 poles (23.1386, -35.8225) (23.0918, -35.7431) (23.0415, -35.6722) (22.9927, -35.6044) knots 4 4 4 4 5 5 5 5
  spline S80 degree 3 poles (22.9927, -35.6044) (22.9877, -35.5976) (22.9826, -35.5908) (22.9776, -35.5841) knots 5 5 5 5 6 6 6 6
  spline S81 degree 3 poles (22.9776, -35.5841) (23.0011, -35.5626) (23.0241, -35.5411) (23.0481, -35.5196) knots 6 6 6 6 7 7 7 7
  spline S82 degree 3 poles (23.0481, -35.5196) (23.0804, -35.4908) (23.1128, -35.462) (23.1462, -35.4332) knots 7 7 7 7 8 8 8 8
  spline S83 degree 3 poles (23.1462, -35.4332) (23.1959, -35.3902) (23.2476, -35.3472) (23.2999, -35.3041) knots 8 8 8 8 9 9 9 9
  spline S84 degree 3 poles (23.2999, -35.3041) (23.3326, -35.2772) (23.3648, -35.2503) (23.3985, -35.2233) knots 9 9 9 9 10 10 10 10
  spline S85 degree 3 poles (23.3985, -35.2233) (23.4577, -35.176) (23.5197, -35.1284) (23.5823, -35.0808) knots 10 10 10 10 11 11 11 11
  spline S86 degree 3 poles (23.5823, -35.0808) (23.6124, -35.0579) (23.6412, -35.0351) (23.6721, -35.0121) knots 11 11 11 11 12 12 12 12
  spline S87 degree 3 poles (23.6721, -35.0121) (23.7669, -34.9414) (23.8649, -34.8704) (23.9677, -34.7986) knots 12 12 12 12 13 13 13 13
  line L15 (23.9677, -34.7986) -> (24.0359, -34.751)
  spline S88 degree 3 poles (24.0359, -34.751) (24.1585, -34.666) (24.2817, -34.5828) (24.4052, -34.502) knots 14 14 14 14 15 15 15 15
  spline S89 degree 3 poles (24.4052, -34.502) (24.5793, -34.3881) (24.7581, -34.2797) (24.9388, -34.1745) knots 15 15 15 15 16 16 16 16
  spline S90 degree 3 poles (24.9388, -34.1745) (24.9699, -34.1564) (25.0007, -34.138) (25.0319, -34.1201) knots 16 16 16 16 17 17 17 17
  ellipse E9 centre (32.057, -38.6381) end of major axis (21.3381, -39.4797) minor radius 6.4317 (25.5636, -33.8342) -> (25.0319, -34.1201) ccw
  spline S91 degree 3 poles (25.5636, -33.8342) (25.5779, -33.827) (25.5924, -33.82) (25.6067, -33.8128) knots 18 18 18 18 19 19 19 19
  spline S92 degree 3 poles (25.6067, -33.8128) (25.6209, -33.9908) (25.6353, -34.1686) (25.6498, -34.3465) knots 19 19 19 19 20 20 20 20
  spline S93 degree 3 poles (25.6498, -34.3465) (25.6701, -34.5958) (25.6904, -34.8452) (25.71, -35.0951) knots 20 20 20 20 21 21 21 21
  arc A0 (25.71, -35.0951) -> (25.7442, -35.5578) centre (-16.7446, -38.4573) cw
  line L16 (25.7442, -35.5578) -> (25.7516, -35.6735)
  spline S94 degree 3 poles (25.7516, -35.6735) (25.7598, -35.7932) (25.7674, -35.9138) (25.7745, -36.0348) knots 23 23 23 23 24 24 24 24
  line L17 (25.7745, -36.0348) -> (25.781, -36.1658)
  spline S95 degree 3 poles (25.781, -36.1658) (25.7872, -36.285) (25.7926, -36.4041) (25.7972, -36.5244) knots 25 25 25 25 26 26 26 26
  line L18 (25.7972, -36.5244) -> (25.8013, -36.6523)
  spline S96 degree 3 poles (25.8013, -36.6523) (25.8053, -36.776) (25.8079, -36.9002) (25.8094, -37.025) knots 27 27 27 27 28 28 28 28
  line L19 (25.8094, -37.025) -> (25.8106, -37.1376)
  spline S97 degree 3 poles (25.8106, -37.1376) (25.812, -37.2732) (25.8106, -37.4091) (25.8086, -37.5429) knots 29 29 29 29 30 30 30 30
  line L20 (25.8086, -37.5429) -> (25.8074, -37.6211)
  spline S98 degree 3 poles (25.8074, -37.6211) (25.8046, -37.7424) (25.8, -37.8601) (25.7944, -37.9762) knots 31 31 31 31 32 32 32 32
  spline S99 degree 3 poles (25.7944, -37.9762) (25.7926, -38.0113) (25.7905, -38.0458) (25.7886, -38.0804) knots 32 32 32 32 33 33 33 33
  spline S100 degree 3 poles (25.7886, -38.0804) (25.7837, -38.1665) (25.7781, -38.2514) (25.7715, -38.335) knots 33 33 33 33 34 34 34 34
  spline S101 degree 3 poles (25.7715, -38.335) (25.7691, -38.3661) (25.7668, -38.3973) (25.7642, -38.4281) knots 34 34 34 34 35 35 35 35
  spline S102 degree 3 poles (25.7642, -38.4281) (25.7545, -38.5405) (25.7437, -38.6515) (25.7308, -38.7605) knots 35 35 35 35 36 36 36 36
  spline S103 degree 3 poles (25.7308, -38.7605) (25.4477, -38.4845) (25.1501, -38.1883) (24.8279, -37.8622) knots 36 36 36 36 37 37 37 37
  ellipse E10 centre (31.448, -24.3019) end of major axis (31.0152, -33.2704) minor radius 5.5772 (27.7173, -17.9148) -> (26.7336, -19.8514) ccw
  spline S104 degree 3 poles (27.7173, -17.9148) (29.0129, -15.9535) (31.1001, -14.3906) (33.5941, -13.5142) knots 1 1 1 1 2 2 2 2
  spline S105 degree 3 poles (33.5941, -13.5142) (38.562, -11.7703) (43.9599, -12.3874) (48.7936, -15.2522) knots 2 2 2 2 3 3 3 3
  ellipse E11 centre (-11.762, -41.0016) end of major axis (-82.0151, -54.8198) minor radius 31.0432 (56.2941, -21.9693) -> (48.7936, -15.2522) ccw
  spline S106 degree 3 poles (56.2941, -21.9693) (56.3974, -22.1233) (56.4992, -22.279) (56.6, -22.4354) knots 4 4 4 4 5 5 5 5
  spline S107 degree 3 poles (56.6, -22.4354) (56.6327, -22.4864) (56.689, -22.5164) (56.7483, -22.5164) (56.7588, -22.5164) (56.7695, -22.5153) (56.7802, -22.5134) knots 5 5 5 5 6 6 6 7 7 7 7
  spline S108 degree 3 poles (56.7802, -22.5134) (61.7783, -21.5941) (68.8966, -20.8717) (72.8262, -21.7919) knots 7 7 7 7 8 8 8 8
  spline S109 degree 3 poles (72.8262, -21.7919) (72.6824, -22.044) (72.686, -22.3861) (72.6889, -22.6745) knots 8 8 8 8 9 9 9 9
  spline S110 degree 3 poles (72.6889, -22.6745) (72.6898, -22.7567) (72.6908, -22.8352) (72.6879, -22.9062) knots 9 9 9 9 10 10 10 10
  spline S111 degree 3 poles (72.6879, -22.9062) (72.6812, -23.0752) (72.6829, -23.2445) (72.6846, -23.4083) knots 10 10 10 10 11 11 11 11
  line L21 (72.6846, -23.4083) -> (72.686, -23.5489)
  spline S112 degree 3 poles (72.686, -23.5489) (72.6889, -23.9602) (72.6367, -24.3483) (72.5816, -24.7593) knots 12 12 12 12 13 13 13 13
  spline S113 degree 3 poles (72.5816, -24.7593) (72.5391, -25.0761) (72.4951, -25.4037) (72.4796, -25.7391) knots 13 13 13 13 14 14 14 14
  spline S114 degree 3 poles (72.4796, -25.7391) (72.4767, -25.8016) (72.4721, -25.8643) (72.4676, -25.9268) knots 14 14 14 14 15 15 15 15
  spline S115 degree 3 poles (72.4676, -25.9268) (72.4454, -26.2291) (72.4204, -26.5695) (72.6009, -26.868) knots 15 15 15 15 16 16 16 16
  spline S116 degree 3 poles (72.6009, -26.868) (71.7537, -26.8572) (70.8866, -26.9583) (70.0455, -27.0555) (69.7444, -27.0902) (69.4457, -27.1249) (69.1506, -27.154) knots 16 16 16 16 17 17 17 18 18 18 18
  spline S117 degree 3 poles (69.1506, -27.154) (67.8344, -27.2846) (66.4945, -27.493) (65.0537, -27.7913) knots 18 18 18 18 19 19 19 19
  spline S118 degree 3 poles (65.0537, -27.7913) (63.4764, -28.1183) (61.7476, -28.5933) (59.769, -29.2434) knots 19 19 19 19 20 20 20 20
  spline S119 degree 3 poles (59.769, -29.2434) (59.6839, -29.2715) (59.6332, -29.3588) (59.6513, -29.4467) knots 20 20 20 20 21 21 21 21
  spline S120 degree 3 poles (59.6513, -29.4467) (59.6587, -29.4824) (59.6668, -29.5178) (59.6749, -29.5528) knots 21 21 21 21 22 22 22 22
  line L22 (59.6749, -29.5528) -> (59.6885, -29.6124)
  spline S121 degree 3 poles (59.6885, -29.6124) (59.7063, -29.692) (59.7762, -29.7492) (59.8578, -29.7506) knots 23 23 23 23 24 24 24 24
  ellipse E12 centre (57.8939, -32.5874) end of major axis (49.8424, -33.2289) minor radius 2.7752 (61.8973, -29.8915) -> (59.8578, -29.7506) ccw
  spline S122 degree 3 poles (61.8973, -29.8915) (64.4124, -30.212) (66.6708, -31.2692) (68.4282, -32.9485) (69.9147, -34.3691) (70.985, -36.1899) (71.5224, -38.2119) knots 25 25 25 25 26 26 26 27 27 27 27
  spline S123 degree 3 poles (71.5224, -38.2119) (71.5769, -38.4276) (71.626, -38.6445) (71.6696, -38.8622) (71.8003, -39.5151) (71.8816, -40.1756) (71.9124, -40.837) knots 27 27 27 27 28 28 28 29 29 29 29
  spline S124 degree 3 poles (71.9124, -40.837) (71.9124, -40.8382) (71.9126, -40.84) (71.9127, -40.842) knots 29 29 29 29 30 30 30 30
  line L23 (71.9127, -40.842) -> (71.9162, -40.9627)
  spline S125 degree 3 poles (71.9162, -40.9627) (71.9441, -41.9977) (71.8413, -43.0497) (71.6104, -44.0892) (70.3297, -49.8559) (64.9307, -52.6344) (61.8267, -53.7774) (61.7659, -53.7998) (61.7223, -53.8537) (61.713, -53.9178) knots 31 31 31 31 32 32 32 33 33 33 34 34 34 34
  ellipse E13 centre (61.8858, -53.9434) end of major axis (61.8306, -53.7767) minor radius 0.1744 (61.713, -53.9178) -> (61.7826, -54.0846) ccw
  spline S126 degree 3 poles (61.7826, -54.0846) (62.4298, -54.565) (63.1965, -54.7821) (64.0081, -55.0119) knots 35 35 35 35 36 36 36 36
  line L24 (64.0081, -55.0119) -> (64.0969, -55.037)
  spline S127 degree 3 poles (64.0969, -55.037) (64.1546, -55.0534) (64.1861, -55.105) (64.1964, -55.1479) knots 37 37 37 37 38 38 38 38
  spline S128 degree 3 poles (64.1964, -55.1479) (64.2035, -55.1766) (64.2083, -55.2313) (64.1633, -55.2732) (63.2917, -56.0864) (61.837, -55.7936) (60.8538, -55.1772) knots 38 38 38 38 39 39 39 40 40 40 40
  ellipse E14 centre (60.7572, -55.3395) end of major axis (60.7989, -55.1545) minor radius 0.1824 (60.8538, -55.1772) -> (60.7138, -55.1564) ccw
  arc A1 (60.7138, -55.1564) -> (60.6035, -55.2452) centre (60.7601, -55.3267) ccw
  spline S129 degree 3 poles (60.6035, -55.2452) (60.5382, -55.371) (60.4628, -55.4745) (60.3737, -55.5609) knots 42 42 42 42 43 43 43 43